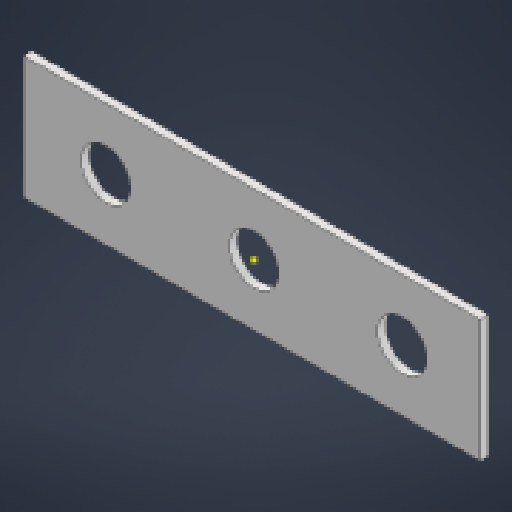
# Autodesk Inventor part: lvl2_2x2_guard
Saved by Autodesk Inventor 2024 (Build 280153000, 153)
## iProperties
Created: 2026-04-08
Part Number: lvl2_2x2_guard
Material: Generic
Document SubType Name: Modeling
Designer: schar
Density: 1 g/cm^3
Appearance: Default
Author: schar
Autodesk Inventor part; units mm, degrees
ref_plane "YZ Plane" through (0, 0, 0) normal (1, 0, 0) x (0, 1, 0)
ref_plane "XZ Plane" through (0, 0, 0) normal (0, 1, 0) x (-1, 0, 0)
ref_plane "XY Plane" through (0, 0, 0) normal (0, 0, 1) x (1, 0, 0)
sketch "Sketch1" plane through (0, 0, 0) normal (0, 0, 1) x (1, 0, 0)
  circle A0 centre (-36.2, 0) radius 6 projected
  circle A1 centre (0, 0) radius 6 projected
  circle A2 centre (36.2, 0) radius 6 projected
  line L0 (-36.2, 0) -> (-18.1, 0)
  line L1 (-36.2, 0) -> (-54.3, 0)
  line L2 (0, 0) -> (18.1, 0)
  line L3 (36.2, 0) -> (54.3, 0)
  line L4 (-54.3, 0) -> (-55.3, 0)
  line L5 (-56.3, 15) -> (-56.3, -15)
  line L6 (-56.3, -15) -> (-54.3, -15)
  line L7 (-54.3, -15) -> (-54.3, 15)
  line L8 (-54.3, 15) -> (-56.3, 15)
  line L9 (-56.3, 15) -> (-54.3, -15) construction
  line L10 (-56.3, -15) -> (-54.3, 15) construction
  line L11 (-19.1, 15) -> (-19.1, -15)
  line L12 (-19.1, -15) -> (-17.1, -15)
  line L13 (-17.1, -15) -> (-17.1, 15)
  line L14 (-17.1, 15) -> (-19.1, 15)
  line L15 (-19.1, 15) -> (-17.1, -15) construction
  line L16 (-19.1, -15) -> (-17.1, 15) construction
  line L17 (17.1, 15) -> (17.1, -15)
  line L18 (17.1, -15) -> (19.1, -15)
  line L19 (19.1, -15) -> (19.1, 15)
  line L20 (19.1, 15) -> (17.1, 15)
  line L21 (17.1, 15) -> (19.1, -15) construction
  line L22 (17.1, -15) -> (19.1, 15) construction
  line L23 (55.3, 15) -> (55.3, -15)
  line L24 (55.3, -15) -> (53.3, -15)
  line L25 (53.3, -15) -> (53.3, 15)
  line L26 (53.3, 15) -> (55.3, 15)
  line L27 (55.3, 15) -> (53.3, -15) construction
  line L28 (55.3, -15) -> (53.3, 15) construction
  line L29 (-56.3, 15) -> (55.3, 15)
  line L30 (55.3, 15) -> (55.3, -15)
  line L31 (55.3, -15) -> (-56.3, -15)
  line L32 (-56.3, -15) -> (-56.3, 15)
  point P0 (0, 0)
  dimension "d0" = 18.1
  dimension "d1" = 18.1
  dimension "d2" = 18.1
  dimension "d3" = 18.1
  dimension "d4" = 1
  dimension "d5" = 30
  dimension "d6" = 2
  dimension "d7" = 30
  dimension "d8" = 2
  dimension "d9" = 2
  constraints: 66 end point, 10 parallel, 8 midpoint, 6 horizontal, 5 perpendicular, 3 vertical
  measures "d0" distance of L0.start L0.end
  measures "d1" distance of L0.start L1.end
  measures "d2" distance of L2.start L2.end
  measures "d3" distance of L3.start L3.end
  measures "d4" distance of L1.end L4.end
  measures "d5" distance of L5.start L5.end
  measures "d6" distance of L12.end L11.end
  measures "d7" distance of L17.start L17.end
  measures "d8" distance of L18.end L17.end
  measures "d9" distance of L23.end L24.end
extrude "Extrusion1" add sketch "Sketch1" along normal blind 2 contours L0 L11 L31 L7 L1 A0 | A0 L1 L7 L29 L11 L0 | L11 L14 L13 L12 | L7 L6 L5 L8 | L29 L17 L31 L13 | L20 L19 L18 L17 | L29 L25 L31 L19 | L26 L23 L24 L25
sketch "Sketch2" plane through (0, 0, 2) normal (0, 0, 1) x (1, 0, 0)
  point P0 (0, 0)
body "Solid1"
